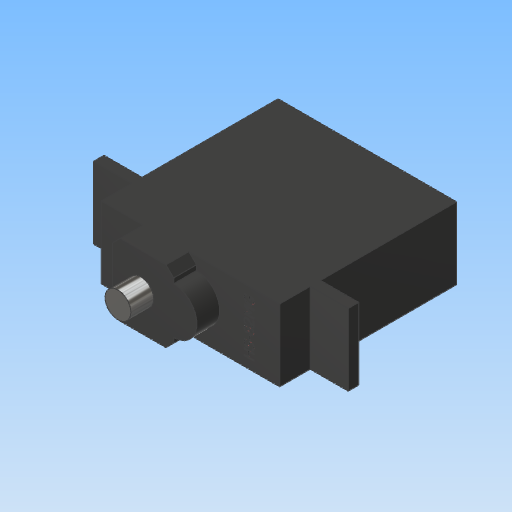
# Autodesk Inventor part: MiniServoBody
Saved by Autodesk Inventor 2017 (Build 210142000, 142)
## iProperties
Created: 2018-04-03
Part Number: MiniServoBody
Material: ABS Plastic
Document SubType Name: Modeling
Designer: Derek Wider
Density: 1.06 g/cm^3
Appearance: Smooth - Black
Author: Derek Wider
Autodesk Inventor part; units mm, degrees
ref_plane "YZ Plane" through (0, 0, 0) normal (1, 0, 0) x (0, 1, 0)
ref_plane "XZ Plane" through (0, 0, 0) normal (0, 1, 0) x (-1, 0, 0)
ref_plane "XY Plane" through (0, 0, 0) normal (0, 0, 1) x (1, 0, 0)
sketch "Sketch1" plane through (0, 0, 0) normal (0, 1, 0) x (-1, 0, 0)
  line L0 (0, 0) -> (29.718, 0)
  line L1 (29.718, 0) -> (29.718, -29.464)
  line L2 (29.718, -29.464) -> (0, -29.464)
  line L3 (0, -29.464) -> (0, 0)
  dimension "d0" = 29.718
  dimension "d1" = 29.464
  constraints: 8 end point, 2 parallel, 1 horizontal, 1 perpendicular
  measures "d0" distance of L1.end L2.end
  measures "d1" distance of L0.end L1.end
extrude "Extrusion1" add sketch "Sketch1" along normal blind 11.938
sketch "Sketch2" plane through (-29.718, 0, 0) normal (0, 0, 1) x (1, 0, 0)
  line L0 (29.718, 0) -> (0, 0) construction
  line L1 (29.718, 0) -> (29.718, 11.938) construction
  line L2 (0, 11.938) -> (29.718, 11.938) construction
  line L3 (0, 0) -> (0, 11.938) construction
  line L4 (0, 11.938) -> (29.718, 11.938) projected
  line L5 (5.715, 11.938) -> (15.875, 11.938)
  line L6 (15.875, 11.938) -> (15.875, 0)
  line L7 (15.875, 0) -> (5.715, 0)
  line L8 (5.715, 0) -> (5.715, 11.938)
  arc A0 (15.875, 2.0927) -> (15.875, 9.8453) centre (15.875, 5.969) ccw
  dimension "d4" = 10.16
  dimension "d5" = 5.715
  constraints: 8 end point, 4 point on line, 2 parallel, 2 point on circle, 1 centre point, 1 coincident, 1 horizontal, 1 line through centre, 1 midpoint, 1 perpendicular
  measures "d4" distance between parallel lines of L8 L6
  measures "d5" distance between parallel lines of L3 L8
extrude "Extrusion2" add sketch "Sketch2" along normal blind 3.81
sketch "Sketch3" plane through (-29.718, 0, 3.81) normal (0, 0, 1) x (1, 0, 0)
  line L0 (5.715, 11.938) -> (5.715, 0) construction
  line L1 (15.875, 11.938) -> (5.715, 11.938) construction
  circle A0 centre (10.414, 5.969) radius 2.159
  line L2 (15.875, 11.938) -> (15.875, 9.8453) projected
  arc A1 (15.875, 2.0927) -> (15.875, 9.8453) centre (15.875, 5.969) ccw projected
  line L3 (15.875, 2.0927) -> (15.875, 0) projected
  line L4 (29.718, 0) -> (15.875, 0) projected
  line L5 (29.718, 0) -> (29.718, 11.938) projected
  line L6 (15.875, 11.938) -> (29.718, 11.938) projected
  dimension "d8" = 4.318
  dimension "d18" = 19.304
  constraints: 1 centre point
  measures "d8" diameter of A0
  measures "d18" distance from line of A0.centre L5
extrude "Extrusion3" add sketch "Sketch3" along normal blind 3.81 contours A0
chamfer "Chamfer1" distance 1.27 angle 45 4 edges at (-24.003, 11.938, 1.905) (-13.843, 11.938, 1.905) (-24.003, 0, 1.905) (-13.843, 0, 1.905)
sketch "Sketch4" plane through (0, 11.938, 0) normal (0, 1, 0) x (1, 0, 0)
  line L0 (-15.113, 0) -> (0, 0) construction
  line L1 (0, 0) -> (0, 29.464) construction
  line L2 (0, 29.464) -> (-29.718, 29.464) construction
  line L3 (-29.718, 29.464) -> (-29.718, 0) construction
  line L4 (-29.718, 0) -> (-22.733, 0) construction
  line L5 (-22.733, -3.81) -> (-22.733, 0) construction
  line L6 (-15.113, -3.81) -> (-22.733, -3.81) construction
  line L7 (-15.113, 0) -> (-15.113, -3.81) construction
  line L8 (-29.718, 5.08) -> (-36.068, 5.08)
  line L9 (-36.068, 5.08) -> (-36.068, 6.8113)
  line L10 (-36.068, 6.8113) -> (-29.718, 6.8113)
  line L11 (-29.718, 6.8113) -> (-29.718, 5.08)
  line L12 (0, 5.08) -> (6.35, 5.08)
  line L13 (6.35, 5.08) -> (6.35, 6.8113)
  line L14 (6.35, 6.8113) -> (0, 6.8113)
  line L15 (0, 6.8113) -> (0, 5.08)
  dimension "d14" = 6.35
  dimension "d15" = 5.08
  constraints: 16 end point, 4 parallel, 4 point on line, 2 horizontal, 2 perpendicular, 1 collinear
  measures "d14" distance of L8.start L8.end
  measures "d15" distance between parallel lines of L8 L4
extrude "Extrusion4" add sketch "Sketch4" against normal up to surface (11.938 mm away)
sketch "Sketch5" plane through (0, 0, 0) normal (0, 0, 1) x (1, 0, 0)
  line L0 (-5.9459, 1.3515) -> (-5.9459, 12.8063) construction
  line L1 (-5.9459, 12.8063) -> (-5.683, 12.8063) construction
  line L2 (-5.683, 12.8063) -> (-5.683, 1.3515) construction
  line L3 (-5.683, 1.3515) -> (-5.9459, 1.3515) construction
  line L4 (-4.2657, 2.7108) -> (-4.2657, 2.4924)
  line L5 (-4.2657, 2.4924) -> (-5.0698, 2.4924)
  line L6 (-5.0698, 2.4924) -> (-5.0698, 1.7362)
  line L7 (-5.0698, 1.7362) -> (-4.2657, 1.7362)
  line L8 (-4.2657, 1.7362) -> (-4.2657, 1.5179)
  line L9 (-4.2657, 1.5179) -> (-5.9086, 1.5179)
  line L10 (-5.9086, 1.5179) -> (-5.9086, 1.7362)
  line L11 (-5.9086, 1.7362) -> (-5.2642, 1.7362)
  line L12 (-5.2642, 1.7362) -> (-5.2642, 2.4924)
  line L13 (-5.2642, 2.4924) -> (-5.9086, 2.4924)
  line L14 (-5.9086, 2.4924) -> (-5.9086, 2.7108)
  line L15 (-5.9086, 2.7108) -> (-4.2657, 2.7108)
  spline S0 degree 2 poles (-4.2364, 3.5016) (-4.2364, 3.3232) (-4.311, 3.0729) (-4.3642, 2.9624) knots 0 0 0 1 2 2 2
  line L16 (-4.3642, 2.9624) -> (-4.6385, 2.9624)
  line L17 (-4.6385, 2.9624) -> (-4.6385, 2.9784)
  spline S1 degree 2 poles (-4.6385, 2.9784) (-4.5373, 3.0862) (-4.4255, 3.3591) (-4.4255, 3.4856) knots 0 0 0 1 2 2 2
  spline S2 degree 2 poles (-4.4255, 3.4856) (-4.4255, 3.6667) (-4.5759, 3.8517) (-4.6997, 3.8517) knots 0 0 0 1 2 2 2
  spline S3 degree 2 poles (-4.6997, 3.8517) (-4.7983, 3.8517) (-4.9207, 3.7545) (-4.9514, 3.6494) knots 0 0 0 1 2 2 2
  spline S4 degree 2 poles (-4.9514, 3.6494) (-4.9727, 3.5735) (-5.0019, 3.447) (-5.0259, 3.3525) knots 0 0 0 1 2 2 2
  spline S5 degree 2 poles (-5.0259, 3.3525) (-5.0485, 3.2673) (-5.1164, 3.1328) (-5.171, 3.0809) knots 0 0 0 1 2 2 2
  spline S6 degree 2 poles (-5.171, 3.0809) (-5.2256, 3.0303) (-5.3721, 2.9744) (-5.4679, 2.9744) knots 0 0 0 1 2 2 2
  spline S7 degree 2 poles (-5.4679, 2.9744) (-5.6676, 2.9744) (-5.9379, 3.2859) (-5.9379, 3.5269) knots 0 0 0 1 2 2 2
  spline S8 degree 2 poles (-5.9379, 3.5269) (-5.9379, 3.6653) (-5.8833, 3.9103) (-5.8314, 4.0155) knots 0 0 0 1 2 2 2
  line L18 (-5.8314, 4.0155) -> (-5.5704, 4.0155)
  line L19 (-5.5704, 4.0155) -> (-5.5704, 3.9995)
  spline S9 degree 2 poles (-5.5704, 3.9995) (-5.6423, 3.921) (-5.7488, 3.676) (-5.7488, 3.5415) knots 0 0 0 1 2 2 2
  spline S10 degree 2 poles (-5.7488, 3.5415) (-5.7488, 3.3898) (-5.6064, 3.202) (-5.4905, 3.202) knots 0 0 0 1 2 2 2
  spline S11 degree 2 poles (-5.4905, 3.202) (-5.3867, 3.202) (-5.2629, 3.3125) (-5.2349, 3.4164) knots 0 0 0 1 2 2 2
  spline S12 degree 2 poles (-5.2349, 3.4164) (-5.2163, 3.4856) (-5.1684, 3.6866) (-5.1484, 3.7532) knots 0 0 0 1 2 2 2
  spline S13 degree 2 poles (-5.1484, 3.7532) (-5.0965, 3.9223) (-4.8875, 4.0794) (-4.7343, 4.0794) knots 0 0 0 1 2 2 2
  spline S14 degree 2 poles (-4.7343, 4.0794) (-4.6372, 4.0794) (-4.4508, 4.0008) (-4.3855, 3.9303) knots 0 0 0 1 2 2 2
  spline S15 degree 2 poles (-4.3855, 3.9303) (-4.3136, 3.8517) (-4.2364, 3.652) (-4.2364, 3.5016) knots 0 0 0 1 2 2 2
  line L20 (-4.8848, 4.8569) -> (-4.8848, 4.2352)
  line L21 (-4.8848, 4.2352) -> (-5.0845, 4.2352)
  line L22 (-5.0845, 4.2352) -> (-5.0845, 4.8569)
  line L23 (-5.0845, 4.8569) -> (-4.8848, 4.8569)
  spline S16 degree 2 poles (-4.2284, 5.5718) (-4.2284, 5.4493) (-4.3017, 5.2483) (-4.3696, 5.1777) knots 0 0 0 1 2 2 2
  spline S17 degree 2 poles (-4.3696, 5.1777) (-4.4361, 5.1085) (-4.6172, 5.0366) (-4.7197, 5.0366) knots 0 0 0 1 2 2 2
  spline S18 degree 2 poles (-4.7197, 5.0366) (-4.8528, 5.0366) (-5.0765, 5.1791) (-5.1431, 5.3149) knots 0 0 0 1 2 2 2
  line L24 (-5.1431, 5.3149) -> (-5.1497, 5.3149)
  spline S19 degree 2 poles (-5.1497, 5.3149) (-5.2203, 5.1937) (-5.388, 5.0766) (-5.5132, 5.0766) knots 0 0 0 1 2 2 2
  spline S20 degree 2 poles (-5.5132, 5.0766) (-5.6982, 5.0766) (-5.9459, 5.3561) (-5.9459, 5.5718) knots 0 0 0 1 2 2 2
  spline S21 degree 2 poles (-5.9459, 5.5718) (-5.9459, 5.7955) (-5.7116, 6.0657) (-5.5278, 6.0657) knots 0 0 0 1 2 2 2
  spline S22 degree 2 poles (-5.5278, 6.0657) (-5.4173, 6.0657) (-5.2016, 5.9366) (-5.1404, 5.8155) knots 0 0 0 1 2 2 2
  line L25 (-5.1404, 5.8155) -> (-5.1338, 5.8155)
  spline S23 degree 2 poles (-5.1338, 5.8155) (-5.0672, 5.9592) (-4.8755, 6.107) (-4.7237, 6.107) knots 0 0 0 1 2 2 2
  spline S24 degree 2 poles (-4.7237, 6.107) (-4.5133, 6.107) (-4.2284, 5.8008) (-4.2284, 5.5718) knots 0 0 0 1 2 2 2
  spline S25 degree 2 poles (-4.7024, 5.8807) (-4.8036, 5.8807) (-4.9234, 5.8008) (-4.9846, 5.6876) knots 0 0 0 1 2 2 2
  spline S26 degree 2 poles (-4.9846, 5.6876) (-5.0059, 5.6504) (-5.0552, 5.5252) (-5.0872, 5.4467) knots 0 0 0 1 2 2 2
  spline S27 degree 2 poles (-5.0872, 5.4467) (-5.0272, 5.3561) (-4.8488, 5.259) (-4.7357, 5.259) knots 0 0 0 1 2 2 2
  spline S28 degree 2 poles (-4.7357, 5.259) (-4.5866, 5.259) (-4.3922, 5.4387) (-4.3922, 5.5745) knots 0 0 0 1 2 2 2
  spline S29 degree 2 poles (-4.3922, 5.5745) (-4.3922, 5.7129) (-4.5586, 5.8807) (-4.7024, 5.8807) knots 0 0 0 1 2 2 2
  spline S30 degree 2 poles (-5.5252, 5.8501) (-5.6357, 5.8501) (-5.7834, 5.7023) (-5.7834, 5.5705) knots 0 0 0 1 2 2 2
  spline S31 degree 2 poles (-5.7834, 5.5705) (-5.7834, 5.4507) (-5.6516, 5.2976) (-5.5385, 5.2976) knots 0 0 0 1 2 2 2
  spline S32 degree 2 poles (-5.5385, 5.2976) (-5.4573, 5.2976) (-5.3441, 5.3761) (-5.2988, 5.4547) knots 0 0 0 1 2 2 2
  spline S33 degree 2 poles (-5.2988, 5.4547) (-5.2802, 5.4879) (-5.215, 5.6291) (-5.1963, 5.6863) knots 0 0 0 1 2 2 2
  spline S34 degree 2 poles (-5.1963, 5.6863) (-5.2695, 5.7822) (-5.4253, 5.8501) (-5.5252, 5.8501) knots 0 0 0 1 2 2 2
  line L26 (-4.2657, 7.3212) -> (-4.2657, 6.3081)
  line L27 (-4.2657, 6.3081) -> (-4.4987, 6.3081)
  spline S35 degree 2 poles (-4.4987, 6.3081) (-4.6012, 6.4172) (-4.7916, 6.6116) (-4.8941, 6.7048) knots 0 0 0 1 2 2 2
  spline S36 degree 2 poles (-4.8941, 6.7048) (-5.1005, 6.8925) (-5.3481, 7.0296) (-5.4799, 7.0296) knots 0 0 0 1 2 2 2
  spline S37 degree 2 poles (-5.4799, 7.0296) (-5.5491, 7.0296) (-5.653, 6.987) (-5.6863, 6.9484) knots 0 0 0 1 2 2 2
  spline S38 degree 2 poles (-5.6863, 6.9484) (-5.7195, 6.9098) (-5.7528, 6.8086) (-5.7528, 6.7474) knots 0 0 0 1 2 2 2
  spline S39 degree 2 poles (-5.7528, 6.7474) (-5.7528, 6.6888) (-5.7235, 6.569) (-5.7009, 6.5144) knots 0 0 0 1 2 2 2
  spline S40 degree 2 poles (-5.7009, 6.5144) (-5.6823, 6.4678) (-5.629, 6.3813) (-5.6104, 6.3546) knots 0 0 0 1 2 2 2
  line L28 (-5.6104, 6.3546) -> (-5.6104, 6.3427)
  line L29 (-5.6104, 6.3427) -> (-5.8447, 6.3427)
  spline S41 degree 2 poles (-5.8447, 6.3427) (-5.878, 6.4106) (-5.9432, 6.6542) (-5.9432, 6.7634) knots 0 0 0 1 2 2 2
  spline S42 degree 2 poles (-5.9432, 6.7634) (-5.9432, 6.9937) (-5.6996, 7.2533) (-5.4919, 7.2533) knots 0 0 0 1 2 2 2
  spline S43 degree 2 poles (-5.4919, 7.2533) (-5.3947, 7.2533) (-5.2323, 7.208) (-5.163, 7.1681) knots 0 0 0 1 2 2 2
  spline S44 degree 2 poles (-5.163, 7.1681) (-5.0911, 7.1282) (-4.95, 7.0123) (-4.8821, 6.9484) knots 0 0 0 1 2 2 2
  spline S45 degree 2 poles (-4.8821, 6.9484) (-4.769, 6.8446) (-4.5267, 6.5903) (-4.4561, 6.5144) knots 0 0 0 1 2 2 2
  line L30 (-4.4561, 6.5144) -> (-4.4561, 7.3212)
  line L31 (-4.4561, 7.3212) -> (-4.2657, 7.3212)
  line L32 (-4.2657, 8.996) -> (-4.2657, 8.7777)
  line L33 (-4.2657, 8.7777) -> (-5.6809, 8.7777)
  line L34 (-5.6809, 8.7777) -> (-4.7184, 8.349)
  line L35 (-4.7184, 8.349) -> (-4.7184, 8.2159)
  line L36 (-4.7184, 8.2159) -> (-5.6809, 7.7912)
  line L37 (-5.6809, 7.7912) -> (-4.2657, 7.7912)
  line L38 (-4.2657, 7.7912) -> (-4.2657, 7.5875)
  line L39 (-4.2657, 7.5875) -> (-5.9086, 7.5875)
  line L40 (-5.9086, 7.5875) -> (-5.9086, 7.8857)
  line L41 (-5.9086, 7.8857) -> (-4.994, 8.2957)
  line L42 (-4.994, 8.2957) -> (-5.9086, 8.6925)
  line L43 (-5.9086, 8.6925) -> (-5.9086, 8.996)
  line L44 (-5.9086, 8.996) -> (-4.2657, 8.996)
  spline S46 degree 2 poles (-4.2338, 10.0172) (-4.2338, 9.8428) (-4.3403, 9.5539) (-4.4481, 9.45) knots 0 0 0 1 2 2 2
  spline S47 degree 2 poles (-4.4481, 9.45) (-4.5573, 9.3462) (-4.8795, 9.2357) (-5.0885, 9.2357) knots 0 0 0 1 2 2 2
  spline S48 degree 2 poles (-5.0885, 9.2357) (-5.2869, 9.2357) (-5.601, 9.3475) (-5.7129, 9.4513) knots 0 0 0 1 2 2 2
  spline S49 degree 2 poles (-5.7129, 9.4513) (-5.8207, 9.5512) (-5.9379, 9.8441) (-5.9379, 10.0185) knots 0 0 0 1 2 2 2
  spline S50 degree 2 poles (-5.9379, 10.0185) (-5.9379, 10.1024) (-5.9139, 10.2541) (-5.8926, 10.3234) knots 0 0 0 1 2 2 2
  spline S51 degree 2 poles (-5.8926, 10.3234) (-5.8766, 10.3793) (-5.8181, 10.5151) (-5.7968, 10.5564) knots 0 0 0 1 2 2 2
  line L45 (-5.7968, 10.5564) -> (-5.5332, 10.5564)
  line L46 (-5.5332, 10.5564) -> (-5.5332, 10.5377)
  spline S52 degree 2 poles (-5.5332, 10.5377) (-5.5691, 10.4964) (-5.6343, 10.4099) (-5.6716, 10.33) knots 0 0 0 1 2 2 2
  spline S53 degree 2 poles (-5.6716, 10.33) (-5.7049, 10.2635) (-5.7488, 10.0917) (-5.7488, 9.9932) knots 0 0 0 1 2 2 2
  spline S54 degree 2 poles (-5.7488, 9.9932) (-5.7488, 9.7562) (-5.392, 9.4633) (-5.0951, 9.4633) knots 0 0 0 1 2 2 2
  spline S55 degree 2 poles (-5.0951, 9.4633) (-4.9301, 9.4633) (-4.6824, 9.5405) (-4.5972, 9.6138) knots 0 0 0 1 2 2 2
  spline S56 degree 2 poles (-4.5972, 9.6138) (-4.512, 9.6843) (-4.4228, 9.884) (-4.4228, 10.0092) knots 0 0 0 1 2 2 2
  spline S57 degree 2 poles (-4.4228, 10.0092) (-4.4228, 10.101) (-4.4494, 10.2848) (-4.4761, 10.3473) knots 0 0 0 1 2 2 2
  line L47 (-4.4761, 10.3473) -> (-4.9008, 10.3473)
  line L48 (-4.9008, 10.3473) -> (-4.9008, 9.9666)
  line L49 (-4.9008, 9.9666) -> (-5.0925, 9.9666)
  line L50 (-5.0925, 9.9666) -> (-5.0925, 10.563)
  line L51 (-5.0925, 10.563) -> (-4.3749, 10.563)
  spline S58 degree 2 poles (-4.3749, 10.563) (-4.3562, 10.5217) (-4.299, 10.3806) (-4.2817, 10.3207) knots 0 0 0 1 2 2 2
  spline S59 degree 2 poles (-4.2817, 10.3207) (-4.2577, 10.2395) (-4.2338, 10.109) (-4.2338, 10.0172) knots 0 0 0 1 2 2 2
  point P0 (0, 0)
  constraints: 2 other
emboss "Emboss1" sketch "Sketch5" operation cut depth 0.254 direction (0, 0, -1)
body "Solid1"
